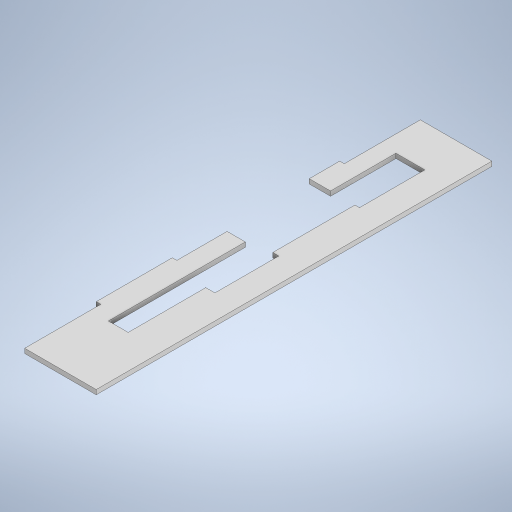
# Autodesk Inventor part: Atas Terminal
Saved by Autodesk Inventor 2024 (Build 280153000, 153)
## iProperties
Created: 2023-08-09
Part Number: Atas Terminal
Material: Generic
Document SubType Name: Modeling
Designer: Asus
Density: 1 g/cm^3
Appearance: Default
Author: Asus
Autodesk Inventor part; units mm, degrees
ref_plane "YZ Plane" through (0, 0, 0) normal (1, 0, 0) x (0, 1, 0)
ref_plane "XZ Plane" through (0, 0, 0) normal (0, 1, 0) x (-1, 0, 0)
ref_plane "XY Plane" through (0, 0, 0) normal (0, 0, 1) x (1, 0, 0)
sketch "Sketch1" plane through (0, 0, 0) normal (0, 1, 0) x (-1, 0, 0)
  line L0 (0, 0) -> (0, -260)
  line L1 (0, -260) -> (47, -260)
  line L2 (47, -260) -> (47, -210)
  line L3 (47, -210) -> (50, -210)
  line L4 (47, -100) -> (50, -100)
  line L5 (50, -100) -> (50, -50)
  line L6 (50, -50) -> (47, -50)
  line L7 (47, -50) -> (47, 0)
  line L8 (47, 0) -> (0, 0)
  line L9 (47, -260) -> (50, -260) construction
  line L10 (50, -260) -> (50, -190) construction
  line L11 (50, -190) -> (35, -190) construction
  line L12 (47, -100) -> (47, -133)
  line L13 (50, -210) -> (50, -190)
  line L14 (47, -260) -> (36, -260) construction
  line L15 (50, -190) -> (47, -190)
  line L16 (36, -260) -> (36, -190) construction
  line L17 (36, -190) -> (36, -233) construction
  line L18 (36, -233) -> (17, -233)
  line L19 (17, -233) -> (17, -190)
  line L20 (17, -190) -> (20, -190)
  line L21 (47, -190) -> (36, -190)
  line L22 (36, -233) -> (36, -190)
  line L23 (47, -133) -> (35, -133) construction
  line L24 (35, -133) -> (35, -43)
  line L25 (35, -43) -> (22, -43)
  line L26 (22, -43) -> (22, -94)
  line L27 (22, -94) -> (16, -94)
  line L28 (16, -94) -> (16, -136)
  line L29 (16, -136) -> (20, -136)
  line L30 (20, -190) -> (20, -136)
  line L31 (47, -133) -> (35, -133)
  dimension "d0" = 260
  dimension "d1" = 47
  dimension "d2" = 50
  dimension "d3" = 3
  dimension "d6" = 50
  dimension "d7" = 70
  dimension "d10" = 11
  dimension "d11" = 27
  dimension "d13" = 43
  dimension "d14" = 19
  dimension "d15" = 12
  dimension "d16" = 90
  dimension "d17" = 13
  dimension "d18" = 51
  dimension "d19" = 6
  dimension "d20" = 42
  constraints: 64 end point, 14 perpendicular, 4 point on line, 3 vertical, 2 collinear, 1 horizontal
  measures "d0" distance of L0.start L0.end
  measures "d1" distance of L0.end L1.end
  measures "d2" distance of L1.end L2.end
  measures "d3" distance of L2.end L3.end
  measures "d6" distance of L4.end L5.end
  measures "d7" distance of L9.end L10.end
  measures "d10" distance of L1.end L14.end
  measures "d11" distance of L15.end L20.end
  measures "d13" distance of L16.end L17.end
  measures "d14" distance of L17.end L18.end
  measures "d15" distance of L12.end L23.end
  measures "d16" distance of L23.end L24.end
  measures "d17" distance of L24.end L25.end
  measures "d18" distance of L25.end L26.end
  measures "d19" distance of L26.end L27.end
  measures "d20" distance of L27.end L28.end
extrude "Extrusion1" add sketch "Sketch1" along normal blind 3
body "Solid1"
